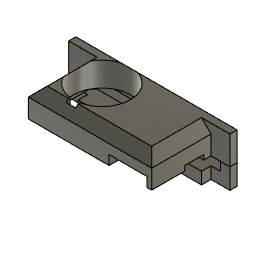
Flashlight Module Cover Plate (Autodesk Fusion 360 design; units mm, degrees)
Autodesk Fusion 360 part; units mm, degrees
sketch "Sketch1" plane through (0, 0, 0) normal (0, 0, 1) x (1, 0, 0)
  line L0 (0, 0) -> (26, 0)
  line L1 (26, 0) -> (26, 14.5)
  line L2 (26, 14.5) -> (0, 14.5)
  line L3 (0, 14.5) -> (0, 0)
  dimension "d1" = 26
  dimension "d2" = 14.5
  constraint horizontal L0
  constraint vertical L1
  constraint horizontal L2
  constraint vertical L3
  constraint coincident L0.start L3.end
  measures "d1" horizontal distance of L0.start L0.end
  measures "d2" vertical distance of L0.start L2.end
sketch "Sketch2" plane through (0, 0, 0) normal (0, 0, 1) x (1, 0, 0)
  line L0 (26, 14.5) -> (0, 14.5)
  line L1 (1, 14.5) -> (1, 1.5)
  line L2 (1, 1.5) -> (14, 1.5)
  line L3 (14, 1.5) -> (14, 14.5)
  line L4 (25, 14.5) -> (25, 11)
  line L5 (25, 11) -> (26, 11)
  line L6 (26, 7) -> (14, 7)
  line L7 (0, 14.5) -> (0, 0)
  line L8 (21, 7) -> (21, 4)
  line L9 (21, 4) -> (25, 4)
  line L10 (25, 4) -> (25, -0.5)
  line L11 (25, -0.5) -> (17, -0.5)
  line L12 (17, -0.5) -> (17, 2.5)
  line L13 (17, 2.5) -> (14, 2.5)
  line L14 (26, 7) -> (26, 11)
  circle A0 centre (7.25, 8.25) radius 6
  line L15 (7.5, 18.5) -> (7.5, -15.5) construction
  line L16 (6.5, 1.5) -> (6.5, 2.2971)
  line L17 (8.5, 1.5) -> (8.5, 2.3817)
  line L18 (26, 0) -> (26, 14.5)
  line L19 (8.5, 1.5) -> (6.5, 1.5)
  line L20 (25, 11) -> (25, 7)
  dimension "d3" = 1
  dimension "d4" = 13
  dimension "d5" = 13
  dimension "d6" = 12
  dimension "d7" = 1
  dimension "d8" = 1
  dimension "d9" = 6.25
  dimension "d10" = 6.25
  dimension "d11" = 1
  dimension "d12" = 3.5
  dimension "d13" = 7.5
  dimension "d14" = 7
  dimension "d15" = 12
  dimension "d16" = 10.5
  dimension "d17" = 4.5
  dimension "d30" = 1
  dimension "d31" = 8
  constraint coincident L0 L1.start
  constraint perpendicular L0 L1
  constraint perpendicular L1 L2
  constraint coincident L0 L3.end
  constraint perpendicular L0 L3
  constraint coincident L0 L4.start
  constraint perpendicular L0 L4
  constraint perpendicular L4 L5
  constraint horizontal L6
  constraint coincident L3 L6.end
  constraint coincident L6 L8.start
  constraint perpendicular L6 L8
  constraint perpendicular L8 L9
  constraint perpendicular L9 L10
  constraint perpendicular L8 L11
  constraint perpendicular L11 L12
  constraint coincident L3 L13.end
  constraint perpendicular L3 L13
  constraint perpendicular L5 L14
  constraint perpendicular L2 L15
  constraint midpoint L2 L15
  constraint coincident L2 L16.start
  constraint perpendicular L2 L16
  constraint coincident L2 L17.start
  constraint perpendicular L2 L17
  constraint coincident A0 L16.end
  constraint coincident A0 L17.end
  constraint coincident L6 L20.end
  constraint perpendicular L6 L20
  measures "d3" distance of L1 L7
  measures "d4" distance of L1 L3
  measures "d5" vertical distance of L1.start L1.end
  measures "d6" diameter of A0
  measures "d7" distance of L15 L16
  measures "d8" distance of L15 L17
  measures "d9" distance of L1 A0.centre
  measures "d10" distance of L0 A0.centre
  measures "d11" distance of L4 L18
  measures "d12" vertical distance of L4.start L4.end
  measures "d13" distance of L0 L6
  measures "d14" distance of L3 L8
  measures "d15" distance of L0 L13
  measures "d16" distance of L0 L9
  measures "d17" distance of L9.end L10.end
  measures "d30" distance of L10 L18
  measures "d31" horizontal distance of L10.end L11.end
extrude "Extrude1" add sketch "Sketch1" along normal blind 6 makes body 1
extrude "Extrude2" cut sketch "Sketch2" along normal blind 0.9 contours L0 L1 L2 L3 A0 L16 L17 bodies 1
extrude "Extrude3" cut sketch "Sketch2" along normal up to surface (6 mm away) contours L2 A0 L16 L17 L19 | A0 bodies 1
extrude "Extrude4" cut sketch "Sketch2" along normal blind 3 contours L0 L3 L4 L6 L20 bodies 1
extrude "Extrude5" cut sketch "Sketch2" along normal blind 1 contours L5 L6 L14 L18 L20 bodies 1
extrude "Extrude6" cut sketch "Sketch2" along normal blind 2 contours L3 L6 L8 L9 L10 L11 L12 L13 bodies 1
sketch "Sketch3" plane through (0, 14.5, 0) normal (0, 1, 0) x (-1, 0, 0)
  line L0 (-25, 0) -> (-25, 3)
  line L1 (-25, 3) -> (-14, 3)
  line L2 (-14, 3) -> (-14, 0.9)
  line L3 (-14, 0.9) -> (-1, 0.9)
  line L4 (-1, 0.9) -> (-1, 0)
  line L5 (-1, 0) -> (0, 0)
  line L6 (0, 0) -> (0, 6)
  line L7 (0, 6) -> (-26, 6)
  line L8 (-26, 6) -> (-26, 0)
  line L9 (-26, 0) -> (-25, 0)
  line L10 (0, 0) -> (-26, 0)
  line L11 (-26, 0) -> (-26, 6)
  line L12 (-26, 6) -> (0, 6)
  line L13 (0, 6) -> (0, 0)
  line L14 (-25, 0) -> (-25, 3)
  line L15 (-25, 3) -> (-14, 3)
  line L16 (-14, 3) -> (-14, 0.9)
  line L17 (-14, 0.9) -> (-1, 0.9)
  line L18 (-1, 0.9) -> (-1, 0)
  line L19 (-1, 0) -> (0, 0)
  line L20 (0, 0) -> (0, 6)
  line L21 (0, 6) -> (-26, 6)
  line L22 (-26, 6) -> (-26, 0)
  line L23 (-26, 0) -> (-25, 0)
  constraint horizontal L10
  constraint vertical L11
  constraint horizontal L12
  constraint vertical L13
  constraint coincident L7.end L8.start
  constraint coincident L5.end L6.start
extrude "Extrude8" add sketch "Sketch3" along normal blind 1.5 bodies 1
sketch "Sketch4" plane through (0, 0, 0) normal (0, 0, -1) x (1, 0, 0)
  line L0 (1, -14.5) -> (1, -1.5)
  line L1 (1, -1.5) -> (14, -1.5)
  line L2 (14, -1.5) -> (14, -2.5)
  line L3 (14, -2.5) -> (17, -2.5)
  line L4 (17, -2.5) -> (17, 0)
  line L5 (17, 0) -> (0, 0)
  line L6 (0, 0) -> (0, -16)
  line L7 (26, -16) -> (0, -16)
  line L8 (0, -16) -> (0, -14.5)
  line L9 (0, -14.5) -> (26, -14.5)
  line L10 (26, -14.5) -> (26, -16)
  line L11 (0, -16) -> (26, -16)
  line L12 (26, -16) -> (26, -11)
  line L13 (26, -11) -> (25, -11)
  line L14 (25, -11) -> (25, -14.5)
  line L15 (25, -14.5) -> (1, -14.5)
  constraint horizontal L7
  constraint vertical L8
  constraint horizontal L9
  constraint vertical L10
  constraint coincident L6 L8.end
  constraint collinear L7 L11
  constraint collinear L9 L15
extrude "Extrude9" add sketch "Sketch4" along normal blind 1.8 contours L6 L7 L8 L9 L10 L11 L12 L15 bodies 1
sketch "Sketch5" plane through (0, 0, -1.8) normal (0, 0, -1) x (1, 0, 0)
  line L0 (0, -16) -> (26, -16)
  line L1 (26, -16) -> (26, -14.5)
  line L2 (26, -14.5) -> (0, -14.5)
  line L3 (0, -14.5) -> (0, -16)
  line L4 (26, -16) -> (0, -16)
  line L5 (0, -16) -> (0, -10.5)
  line L6 (0, -10.5) -> (26, -10.5)
  line L7 (26, -10.5) -> (26, -16)
  line L8 (0, -14.5) -> (0, 0)
  dimension "d38" = 5.5
  constraint horizontal L4
  constraint vertical L5
  constraint horizontal L6
  constraint vertical L7
  constraint coincident L5.end L8
  constraint coincident L0.end L1.start
  measures "d38" distance of L0.start L5.end
extrude "Extrude10" add sketch "Sketch5" along normal blind 2.5 bodies 1
sketch "Sketch6" plane through (0, 0, 6) normal (0, 0, 1) x (-1, 0, 0)
  line L0 (-8.5, -1.5) -> (-6.5, -1.5)
  line L1 (-6.5, -1.5) -> (-6.5, -2.2971)
  arc A0 (-8.5, -2.3817) -> (-6.5, -2.2971) centre (-7.25, -8.25) ccw
  line L2 (-8.5, -2.3817) -> (-8.5, -1.5)
  line L3 (0, -16) -> (0, 0)
  line L4 (0, 0) -> (-26, 0)
  line L5 (-26, 0) -> (-26, -16)
  line L6 (-26, -16) -> (0, -16)
  line L7 (0, -16) -> (4, -16)
  line L8 (4, -16) -> (4, -12.5)
  line L9 (4, -12.5) -> (0, -12.5)
  line L10 (0, -12.5) -> (0, -16)
  line L11 (0, -14.5) -> (-1, -14.5)
  line L12 (0, -14.5) -> (2, -12.5)
  line L13 (-13, -27.3886) -> (-13, -4.6114) construction
  line L14 (-26, -16) -> (-30, -16)
  line L15 (-30, -16) -> (-30, -12.5)
  line L16 (-30, -12.5) -> (-26, -12.5)
  line L17 (-26, -14.5) -> (-28, -12.5)
  line L18 (-26, -12.5) -> (-26, -16)
  dimension "d41" = 45
  dimension "d42" = 4
  dimension "d43" = 3.5
  constraint horizontal L7
  constraint vertical L8
  constraint horizontal L9
  constraint vertical L10
  constraint coincident L3.start L6.end
  constraint coincident L11.start L12.start
  constraint coincident L9 L12.end
  constraint vertical L13
  constraint midpoint L6 L13
  constraint symmetric L3.start L13 L5.end
  constraint symmetric L7.end L13 L14.end
  constraint symmetric L8.end L13 L15.end
  constraint symmetric L9.end L13 L16.end
  constraint symmetric L11.start L13 L17.start
  constraint symmetric L12.end L13 L17.end
  measures "d41" angle of L10 L12
  measures "d42" distance of L3.start L7.end
  measures "d43" distance of L7.end L8.end
extrude "Extrude11" add sketch "Sketch6" against normal up to surface (10.3 mm away) contours L3 L7 L8 L9 L10 L12 | L3 L9 L10 L12 | L5 L14 L15 L16 L17 L18 | L5 L16 L17 L18 bodies 1
extrude "Extrude12" cut sketch "Sketch6" against normal up to surface (1.8 mm away) from surface at -6 contours L3 L9 L10 L12 | L5 L16 L17 L18 bodies 1
chamfer "Chamfer1" distance 2 angle 45 7 edges at (-4, 16, 0.85) (30, 16, 0.85) (13, 16, -4.3) (13, 16, 6) (26, 6.25, 6) (13, 0, 6) (0, 6.25, 6) on bodies 1
split "Split1" by plane through (0, 0, 0) normal (0, 0, -1) bodies 1 makes body 2 at (8.6667, 13.8333, -1.8)
